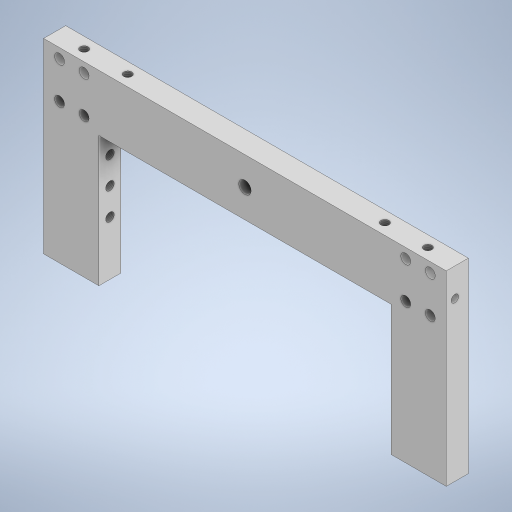
# Autodesk Inventor part: 1-18 hudson
Saved by Autodesk Inventor 2024.2 (Build 282272000, 272)
## iProperties
Created: 2024-11-01
Part Number: 1-18 hudson
Material: Generic
Document SubType Name: Modeling
Designer: Jimena Brenes
Density: 1 g/cm^3
Appearance: Default
Author: Jimena Brenes
Autodesk Inventor part; units mm, degrees
ref_plane "YZ Plane" through (0, 0, 0) normal (1, 0, 0) x (0, 1, 0)
ref_plane "XZ Plane" through (0, 0, 0) normal (0, 1, 0) x (-1, 0, 0)
ref_plane "XY Plane" through (0, 0, 0) normal (0, 0, 1) x (1, 0, 0)
sketch "Sketch1" plane through (0, 0, 0) normal (0, 0, 1) x (1, 0, 0)
  line L0 (0, 0) -> (164, 0)
  line L1 (164, 0) -> (164, -23)
  line L2 (164, -23) -> (0, -23)
  line L3 (0, -23) -> (0, 0)
  line L4 (0, -23) -> (22.5, -23)
  line L5 (22.5, -23) -> (22.5, -76)
  line L6 (22.5, -76) -> (0, -76)
  line L7 (0, -76) -> (0, -23)
  line L8 (164, -23) -> (141.5, -23)
  line L9 (141.5, -23) -> (141.5, -76)
  line L10 (141.5, -76) -> (164, -76)
  line L11 (164, -76) -> (164, -23)
  dimension "d0" = 164
  dimension "d1" = 23
  dimension "d2" = 53
  dimension "d3" = 53
  dimension "d4" = 22.5
  dimension "d5" = 22.5
  constraints: 24 end point, 6 parallel, 3 horizontal, 3 perpendicular
  measures "d0" distance between parallel lines of L1 L3
  measures "d1" distance between parallel lines of L2 L0
  measures "d2" distance between parallel lines of L6 L2
  measures "d3" distance between parallel lines of L2 L10
  measures "d4" distance between parallel lines of L7 L5
  measures "d5" distance between parallel lines of L11 L9
extrude "Extrusion1" add sketch "Sketch1" along normal blind 9
sketch "Sketch2" plane through (0, 0, 9) normal (0, 0, 1) x (1, 0, 0)
  line L0 (6.5, -4) -> (16.5, -4) construction
  line L1 (16.5, -4) -> (16.5, -19) construction
  line L2 (16.5, -19) -> (6.5, -19) construction
  line L3 (6.5, -19) -> (6.5, -4) construction
  line L4 (147.5, -4) -> (157.5, -4) construction
  line L5 (157.5, -4) -> (157.5, -19) construction
  line L6 (157.5, -19) -> (147.5, -19) construction
  line L7 (147.5, -19) -> (147.5, -4) construction
  circle A0 centre (16.5, -4) radius 2
  circle A1 centre (6.5, -4) radius 2
  circle A2 centre (6.5, -19) radius 2
  circle A3 centre (16.5, -19) radius 2
  line L8 (0, 0) -> (0, -76) projected
  line L9 (164, 0) -> (0, 0) projected
  line L10 (22.5, -23) -> (141.5, -23) projected
  line L11 (164, -76) -> (164, 0) projected
  circle A4 centre (157.5, -4) radius 2
  circle A5 centre (157.5, -19) radius 2
  circle A6 centre (147.5, -19) radius 2
  circle A7 centre (147.5, -4) radius 2
  circle A8 centre (82, -11.5) radius 2.5
  dimension "d8" = 4
  dimension "d9" = 4
  dimension "d10" = 4
  dimension "d11" = 4
  dimension "d12" = 6.5
  dimension "d13" = 10
  dimension "d14" = 4
  dimension "d15" = 4
  dimension "d16" = 6.5
  dimension "d17" = 4
  dimension "d18" = 10
  dimension "d19" = 4
  dimension "d20" = 4
  dimension "d21" = 4
  dimension "d22" = 4
  dimension "d23" = 5
  dimension "d24" = 65.5
  dimension "d25" = 11.5
  constraints: 16 end point, 9 centre point, 8 coincident, 4 parallel, 2 horizontal, 2 perpendicular, 2 point on line
  measures "d8" diameter of A0
  measures "d9" diameter of A1
  measures "d10" diameter of A2
  measures "d11" diameter of A3
  measures "d12" distance between parallel lines of L8 L3
  measures "d13" distance between parallel lines of L3 L1
  measures "d14" distance between parallel lines of L9 L0
  measures "d15" distance between parallel lines of L10 L2
  measures "d16" distance between parallel lines of L11 L5
  measures "d17" distance between parallel lines of L10 L6
  measures "d18" distance between parallel lines of L5 L7
  measures "d19" diameter of A4
  measures "d20" diameter of A5
  measures "d21" diameter of A6
  measures "d22" diameter of A7
  measures "d23" diameter of A8
  measures "d24" horizontal distance of L4.start A8.centre
  measures "d25" distance from line of L9 A8.centre
hole "Hole1" at (6.5, -4, 9) at (16.5, -4, 9) at (16.5, -19, 9) at (6.5, -19, 9) at (147.5, -4, 9) at (147.5, -19, 9) at (157.5, -19, 9) at (157.5, -4, 9) direction (0, 0, -1) diameter 4 end through all
hole "Hole2" at (82, -11.5, 9) direction (0, 0, -1) diameter 5 end through all
sketch "Sketch3" plane through (0, 0, 0) normal (0, 1, 0) x (1, 0, 0)
  line L0 (12, -4.5) -> (29.75, -4.5) construction
  circle A0 centre (12, -4.5) radius 2
  circle A1 centre (29.75, -4.5) radius 2
  line L1 (0, 0) -> (0, -9) projected
  line L2 (164, -9) -> (0, -9) projected
  line L3 (134.5, -4.5) -> (152, -4.5) construction
  circle A2 centre (152, -4.5) radius 2
  circle A3 centre (134.5, -4.5) radius 2
  line L4 (164, 0) -> (164, -9) projected
  dimension "d40" = 4
  dimension "d41" = 4
  dimension "d42" = 17.75
  dimension "d43" = 12
  dimension "d44" = 4.5
  dimension "d45" = 4
  dimension "d46" = 4
  dimension "d47" = 17.5
  dimension "d48" = 4.5
  dimension "d49" = 12
  constraints: 4 centre point, 4 coincident, 4 end point, 2 horizontal
  measures "d40" diameter of A0
  measures "d41" diameter of A1
  measures "d42" distance of L0.start L0.end
  measures "d43" distance from line of L1 L0.start
  measures "d44" distance between parallel lines of L2 L0
  measures "d45" diameter of A2
  measures "d46" diameter of A3
  measures "d47" distance of L3.start L3.end
  measures "d48" distance between parallel lines of L2 L3
  measures "d49" distance from line of L4 L3.end
hole "Hole3" at (134.5, 0, 4.5) at (29.75, 0, 4.5) direction (0, -1, 0) diameter 3.242 depth 10 tip angle 118 thread size "M4x0.7" class "6H" standard "ANSI Metric M Profile"
hole "Hole4" at (12, 0, 4.5) at (152, 0, 4.5) direction (0, -1, 0) diameter 3.242 depth 31 tip angle 118 thread size "M4x0.7" class "6H" standard "ANSI Metric M Profile"
sketch "Sketch4" plane through (0, -76, 0) normal (0, -1, 0) x (1, 0, 0)
  circle A0 centre (12, 4.5) radius 2
  line L0 (0, 0) -> (0, 9) projected
  line L1 (0, 9) -> (22.5, 9) projected
  circle A1 centre (152, 4.5) radius 2
  line L2 (141.5, 9) -> (164, 9) projected
  line L3 (164, 0) -> (164, 9) projected
  dimension "d64" = 4
  dimension "d65" = 12
  dimension "d66" = 4.5
  dimension "d67" = 4
  dimension "d68" = 4.5
  dimension "d69" = 12
  constraints: 2 centre point
  measures "d64" diameter of A0
  measures "d65" distance from line of L0 A0.centre
  measures "d66" distance from line of L1 A0.centre
  measures "d67" diameter of A1
  measures "d68" distance from line of L2 A1.centre
  measures "d69" distance from line of L3 A1.centre
hole "Hole5" at (12, -76, 4.5) at (152, -76, 4.5) direction (0, 1, 0) diameter 3.242 depth 10 tip angle 118 thread size "M4x0.7" class "6H" standard "ANSI Metric M Profile"
sketch "Sketch6" plane through (0, -76, 0) normal (-1, 0, 0) x (0, 0, 1)
  line L0 (4.5, 44) -> (4.5, 22) construction
  circle A0 centre (4.5, 44) radius 2
  circle A1 centre (4.5, 33) radius 2
  circle A2 centre (4.5, 22) radius 2
  line L1 (0, 76) -> (0, 0) projected
  line L2 (0, 0) -> (9, 0) projected
  circle A3 centre (3.5, 64.5) radius 1.5
  line L3 (9, 76) -> (9, 0) projected
  line L4 (0, 76) -> (9, 76) projected
  dimension "d83" = 4
  dimension "d84" = 4
  dimension "d85" = 4
  dimension "d86" = 4.5
  dimension "d87" = 22
  dimension "d88" = 11
  dimension "d89" = 3
  dimension "d90" = 5.5
  dimension "d91" = 11.5
  constraints: 4 centre point, 2 coincident, 2 end point, 1 midpoint, 1 vertical
  measures "d83" diameter of A0
  measures "d84" diameter of A1
  measures "d85" diameter of A2
  measures "d86" distance between parallel lines of L1 L0
  measures "d87" distance from line of L2 L0.end
  measures "d88" distance of L0.end A1.centre
  measures "d89" diameter of A3
  measures "d90" distance from line of L3 A3.centre
  measures "d91" distance from line of L4 A3.centre
hole "Hole7" at (0, -11.5, 3.5) direction (1, 0, 0) diameter 3 depth 6 tip angle 118
sketch "Sketch7" plane through (164, -76, 0) normal (1, 0, 0) x (0, 0, -1)
  line L0 (-4.5, 22) -> (-4.5, 44) construction
  circle A0 centre (-4.5, 44) radius 2
  circle A1 centre (-4.5, 22) radius 2
  line L1 (0, 0) -> (0, 76) projected
  line L2 (0, 0) -> (-9, 0) projected
  circle A2 centre (-4.5, 33) radius 2
  circle A3 centre (-5.5, 64.5) radius 1.5
  line L3 (0, 76) -> (-9, 76) projected
  dimension "d106" = 4
  dimension "d108" = 4
  dimension "d109" = 4.5
  dimension "d110" = 22
  dimension "d111" = 4
  dimension "d112" = 11
  dimension "d113" = 3
  dimension "d114" = 5.5
  dimension "d115" = 11.5
  constraints: 4 centre point, 2 coincident, 2 end point, 1 midpoint, 1 vertical
  measures "d106" diameter of A0
  measures "d108" diameter of A1
  measures "d109" distance between parallel lines of L1 L0
  measures "d110" distance from line of L2 L0.start
  measures "d111" diameter of A2
  measures "d112" distance of L0.start A2.centre
  measures "d113" diameter of A3
  measures "d114" distance from line of L1 A3.centre
  measures "d115" distance from line of L3 A3.centre
hole "Hole9" at (164, -11.5, 5.5) direction (-1, 0, 0) diameter 3 depth 10 tip angle 118
sketch "Sketch8" plane through (22.5, -76, 0) normal (1, 0, 0) x (0, 0, -1)
  circle A0 centre (-4.5, 44) radius 1.7294 projected
  line L0 (-9, 76) -> (-9, 0) projected
  circle A1 centre (-4.5, 44) radius 1.7294
  circle A2 centre (-4.5, 33) radius 1.7294 projected
  circle A3 centre (-4.5, 33) radius 2
  circle A4 centre (-4.5, 22) radius 1.7294 projected
  circle A5 centre (-4.5, 22) radius 2
  point P0 (0, 76)
  dimension "d130" = 4
  dimension "d131" = 4
  constraints: 3 centre point, 3 coincident, 1 concentric
  measures "d130" diameter of A3
  measures "d131" diameter of A5
hole "Hole10" at (22.5, -32, 4.5) at (22.5, -43, 4.5) at (22.5, -54, 4.5) direction (-1, 0, 0) diameter 3.4587 depth 10 tip angle 118 thread size "M4x0.5" class "6H" standard "ANSI Metric M Profile"
sketch "Sketch9" plane through (141.5, -76, 0) normal (-1, 0, 0) x (0, 0, 1)
  line L0 (4.5, 44) -> (4.5, 22) construction
  circle A0 centre (4.5, 44) radius 2
  circle A1 centre (4.5, 33) radius 2
  circle A2 centre (4.5, 22) radius 2
  line L1 (9, 0) -> (9, 76) projected
  line L2 (0, 0) -> (9, 0) projected
  point P0 (0, 76)
  dimension "d139" = 4
  dimension "d140" = 4
  dimension "d141" = 4
  dimension "d142" = 4.5
  dimension "d143" = 11
  dimension "d144" = 22
  dimension "d145" = 11
  constraints: 3 centre point, 2 coincident, 2 end point, 1 midpoint, 1 vertical
  measures "d139" diameter of A0
  measures "d140" diameter of A1
  measures "d141" diameter of A2
  measures "d142" distance between parallel lines of L1 L0
  measures "d143" distance of A1.centre L0.end
  measures "d144" distance from line of L2 L0.end
  measures "d145" distance of A1.centre L0.start
hole "Hole11" at (141.5, -32, 4.5) at (141.5, -43, 4.5) at (141.5, -54, 4.5) direction (1, 0, 0) diameter 3.4587 depth 10 tip angle 118 thread size "M4x0.5" class "6H" standard "ANSI Metric M Profile"
equation "\"d5\" = d4"
body "Solid1"
